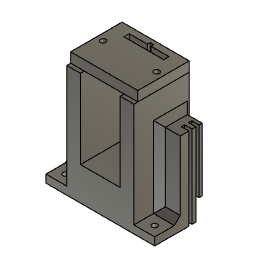
NeckServoMount v8 (Autodesk Fusion 360 design; units mm, degrees)
Autodesk Fusion 360 part; units mm, degrees
sketch "Base" plane through (0, 0, 0) normal (0, 0, 1) x (1, 0, 0) in component "NeckServoMount"
  line L0 (0, 0) -> (55.4, 0)
  line L1 (55.4, 0) -> (55.4, 24.2)
  line L2 (55.4, 24.2) -> (0, 24.2)
  line L3 (0, 24.2) -> (0, 0)
  line L4 (0, 13) -> (55.4, 13)
  line L5 (0, 19) -> (55.4, 19) construction
  line L6 (0, 17.4) -> (55.4, 17.4) construction
  line L7 (0, 21) -> (55.4, 21) construction
  line L8 (0, 22.6) -> (55.4, 22.6) construction
  line L9 (3.8, 22.6) -> (3.8, 21)
  line L10 (3.8, 19) -> (3.8, 17.4)
  line L11 (0, 22.6) -> (3.8, 22.6)
  line L12 (3.8, 21) -> (0, 21)
  line L13 (0, 19) -> (3.8, 19)
  line L14 (0, 17.4) -> (3.8, 17.4)
  line L15 (27.7, 24.2) -> (27.7, 0) construction
  line L16 (55.4, 22.6) -> (51.6, 22.6)
  line L17 (51.6, 22.6) -> (51.6, 21)
  line L18 (51.6, 21) -> (55.4, 21)
  line L19 (51.6, 19) -> (51.6, 17.4)
  line L20 (55.4, 19) -> (51.6, 19)
  line L21 (55.4, 17.4) -> (51.6, 17.4)
  dimension "d1" = 55.4
  dimension "d3" = 13
  dimension "d4" = 4.4
  dimension "d5" = 1.6
  dimension "d6" = 2
  dimension "d7" = 1.6
  dimension "d8" = 1.6
  dimension "d9" = 3.8
  constraint horizontal L0
  constraint vertical L1
  constraint horizontal L2
  constraint vertical L3
  constraint coincident L0.start L3.end
  constraint coincident L3 L4.start
  constraint coincident L1 L4.end
  constraint perpendicular L1 L4
  constraint coincident L3 L5.start
  constraint coincident L1 L5.end
  constraint perpendicular L1 L5
  constraint coincident L3 L6.start
  constraint coincident L1 L6.end
  constraint perpendicular L1 L6
  constraint coincident L3 L7.start
  constraint coincident L1 L7.end
  constraint perpendicular L1 L7
  constraint coincident L3 L8.start
  constraint coincident L1 L8.end
  constraint perpendicular L1 L8
  constraint coincident L8 L9.start
  constraint coincident L7 L9.end
  constraint perpendicular L7 L9
  constraint coincident L5 L10.start
  constraint coincident L6 L10.end
  constraint perpendicular L6 L10
  constraint collinear L9 L10
  constraint midpoint L2 L15.start
  constraint midpoint L0 L15.end
  constraint symmetric L5.start L15 L5.end
  constraint symmetric L6.start L15 L6.end
  constraint symmetric L7.start L15 L7.end
  constraint symmetric L8.start L15 L8.end
  constraint symmetric L9.start L15 L16.end
  constraint symmetric L9.end L15 L17.end
  constraint symmetric L10.start L15 L19.start
  constraint symmetric L10.end L15 L19.end
  measures "d1" distance of L0.start L0.end
  measures "d3" distance of L0 L4
  measures "d4" distance of L4 L6
  measures "d5" distance of L5 L6
  measures "d6" distance of L5 L7
  measures "d7" distance of L7 L8
  measures "d8" distance of L2 L8
  measures "d9" distance of L3 L9
extrude "ExtrudeSlottedVertical" add sketch "Base" along normal blind 42 contours L1 L2 L3 L4 L9 L10 L11 L12 L13 L14 L16 L17 L18 L19 L20 L21 makes body 1 in component "NeckServoMount"
extrude "ExtrudeBasePlate" add sketch "Base" along normal blind 4 contours L0 L1 L3 L4 bodies 1 in component "NeckServoMount"
sketch "Back" plane through (0, 24.2, 0) normal (0, 1, 0) x (-1, 0, 0) in component "NeckServoMount"
  line L0 (-55.4, 0) -> (0, 0)
  line L1 (0, 0) -> (0, 42)
  line L2 (0, 42) -> (-55.4, 42)
  line L3 (-55.4, 42) -> (-55.4, 0)
  line L4 (-55.4, 0) -> (0.6, 0)
  line L5 (0.6, 0) -> (0.6, 10)
  line L6 (0.6, 10) -> (-55.4, 10)
  line L7 (-55.4, 10) -> (-55.4, 0)
  dimension "d19" = 10
  constraint horizontal L4
  constraint vertical L5
  constraint horizontal L6
  constraint vertical L7
  constraint coincident L0.start L3.end
  measures "d19" distance of L0.start L6.end
extrude "CutBackAway" cut sketch "Back" against normal up to surface (3.2 mm away) contours L0 L1 L3 L4 L6 L7 bodies 1 in component "NeckServoMount"
chamfer "Chamfer1" distance 3 angle 45 1 edges at (27.7, 13, 4) on bodies 1 in component "NeckServoMount"
sketch "ScrewHoles" plane through (0, 0, 4) normal (0, 0, 1) x (-1, 0, 0) in component "NeckServoMount"
  line L0 (-55.4, -10) -> (0, -10)
  line L1 (0, -10) -> (0, 0)
  line L2 (0, 0) -> (-55.4, 0)
  line L3 (-55.4, 0) -> (-55.4, -10)
  line L4 (0, -5) -> (-55.4, -5) construction
  circle A0 centre (-5, -5) radius 1.4
  line L5 (-27.7, 0) -> (-27.7, -10) construction
  circle A1 centre (-50.4, -5) radius 1.4
  dimension "d23" = 2.8
  dimension "d49" = 5
  constraint midpoint L1 L4.start
  constraint midpoint L3 L4.end
  constraint coincident L4 A0.centre
  constraint midpoint L2 L5.start
  constraint midpoint L0 L5.end
  constraint symmetric A0 L5 A1
  measures "d23" diameter of A0
  measures "d49" distance of L1 A0.centre
extrude "CutScrewHoles" cut sketch "ScrewHoles" against normal up to surface (4 mm away) contours A0 | A1 bodies 1 in component "NeckServoMount"
sketch "ServoU" plane through (0, 24.2, 0) normal (0, 1, 0) x (-1, 0, 0) in component "NeckServoMount"
  line L0 (-55.4, 10) -> (0, 10)
  line L1 (0, 10) -> (0, 42)
  line L2 (0, 42) -> (-55.4, 42)
  line L3 (-55.4, 42) -> (-55.4, 10)
  line L4 (0, 0) -> (-55.4, 0)
  line L5 (-37.8, 57.2) -> (-17.6, 57.2)
  line L6 (-17.6, 57.2) -> (-17.6, 17)
  line L7 (-17.6, 17) -> (-37.8, 17)
  line L8 (-37.8, 17) -> (-37.8, 57.2)
  line L9 (-10.6, 57.2) -> (-10.6, 3)
  line L10 (-44.8, 57.2) -> (-44.8, 3)
  line L11 (-44.8, 3) -> (-10.6, 3)
  line L12 (-10.6, 57.2) -> (-17.6, 57.2)
  line L13 (-37.8, 57.2) -> (-44.8, 57.2)
  point P0 (-10.6, 57.2)
  point P1 (-44.8, 57.2)
  dimension "d26" = 20.2
  dimension "d27" = 40.2
  dimension "d29" = 17.6
  dimension "d31" = 17
  dimension "d34" = 7
  dimension "d35" = 7
  dimension "d36" = 14
  constraint horizontal L5
  constraint vertical L6
  constraint horizontal L7
  constraint vertical L8
  constraint horizontal L5.start P1
  constraint horizontal P0 P1
  constraint coincident P0 L9.start
  constraint perpendicular L4 L9
  constraint coincident P1 L10.start
  constraint perpendicular L4 L10
  constraint horizontal L9.end L10.end
  measures "d26" distance of L5.start L5.end
  measures "d27" distance of L5.start L7.end
  measures "d29" distance of L3 L8
  measures "d31" distance of L4 L7
  measures "d34" distance of L8 P1
  measures "d35" distance of L6 P0
  measures "d36" distance of L7 L11
extrude "ExtrudeServoU" add sketch "ServoU" against normal up to surface (22.2 mm away) from surface at -2 contours L0 L2 L6 L7 L8 L9 L10 | L0 L9 L10 L11 | L2 L8 L10 L13 | L2 L6 L9 L12 bodies 1 in component "NeckServoMount"
extrude "CutServoU" cut sketch "ServoU" against normal blind 2 contours L0 L2 L6 L7 L8 L9 L10 | L0 L9 L10 L11 | L2 L8 L10 L13 | L2 L6 L9 L12 bodies 1 in component "NeckServoMount"
extrude "CutServoU2" cut sketch "ServoU" against normal through all contours L2 L5 L6 L8 | L2 L6 L7 L8 bodies 1 in component "NeckServoMount"
extrude "CutBackAwayAgain" cut sketch "Back" against normal up to surface (3.2 mm away) contours L0 L1 L3 L4 L6 L7 bodies 1 in component "NeckServoMount"
sketch "BottomSlot" plane through (0, 0, 17) normal (0, 0, 1) x (-1, 0, 0) in component "NeckServoMount"
  line L0 (-17.6, -22.2) -> (-17.6, 0)
  line L1 (-17.6, 0) -> (-37.8, 0)
  line L2 (-37.8, 0) -> (-37.8, -22.2)
  line L3 (-37.8, -22.2) -> (-17.6, -22.2)
  line L4 (-17.6, -22.2) -> (-37.8, -22.2)
  line L5 (-37.8, -22.2) -> (-37.8, -24.9)
  line L6 (-37.8, -24.9) -> (-17.6, -24.9)
  line L7 (-17.6, -24.9) -> (-17.6, -22.2)
  dimension "d54" = 2.7
  dimension "d55" = 20.2
  constraint horizontal L4
  constraint vertical L5
  constraint horizontal L6
  constraint vertical L7
  constraint coincident L0.start L3.end
  measures "d54" distance of L0.start L6.end
  measures "d55" distance of L5 L7
extrude "ExtrudeSlotHolder" add 1 faces at (15.2667, 22.2, 38.7333) along direction (0, 1, 0) blind 6 on bodies 1 bodies 1 in component "NeckServoMount"
extrude "CutBottomSlot" cut sketch "BottomSlot" against normal up to surface (7 mm away) contours L3 L4 L5 L6 L7 bodies 1 in component "NeckServoMount"
sketch "TinySlot" plane through (0, 24.9, 0) normal (0, -1, 0) x (1, 0, 0)
  line L0 (17.6, 10) -> (37.8, 10)
  line L1 (37.8, 10) -> (37.8, 17)
  line L2 (37.8, 17) -> (17.6, 17)
  line L3 (17.6, 17) -> (17.6, 10)
  line L4 (26.8, 17) -> (28.6, 17)
  line L5 (28.6, 17) -> (28.6, 10)
  line L6 (28.6, 10) -> (26.8, 10)
  line L7 (26.8, 10) -> (26.8, 17)
  point P0 (27.7, 17)
  point P1 (27.7, 17)
  dimension "d61" = 1.8
  dimension "d62" = 7
  constraint horizontal L4
  constraint vertical L5
  constraint horizontal L6
  constraint vertical L7
  constraint coincident L2 L4.start
  constraint midpoint L2 P1
  constraint midpoint L4 P1
  constraint coincident P1 P0
  measures "d61" distance of L4.start L4.end
  measures "d62" distance of L4.start L6.end
extrude "CutTinySlot" cut sketch "TinySlot" against normal blind 1.4 contours L0 L2 L4 L5 L6 L7 bodies 1 in component "NeckServoMount"
sketch "TopPlate" plane through (0, 0, 57.2) normal (0, 0, 1) x (-1, 0, 0) in component "TopPlate"
  line L0 (-10.6, 0) -> (-17.6, 0)
  line L1 (-17.6, 0) -> (-17.6, -28.2)
  line L2 (-17.6, -28.2) -> (-10.6, -28.2)
  line L3 (-10.6, -28.2) -> (-10.6, 0)
  line L4 (-10.6, -28.2) -> (-44.8, -28.2)
  line L5 (-44.8, -28.2) -> (-44.8, -2)
  line L6 (-44.8, -2) -> (-10.6, -2)
  line L7 (-10.6, -2) -> (-10.6, -28.2)
  line L8 (-44.8, -10) -> (-44.8, 0)
  line L9 (-17.6, -24.9) -> (-26.8, -24.9)
  line L10 (-37.8, -22.2) -> (-17.6, -22.2)
  line L11 (-26.8, -24.9) -> (-26.8, -26.3)
  line L12 (-26.8, -26.3) -> (-28.6, -26.3)
  line L13 (-28.6, -26.3) -> (-28.6, -24.9)
  line L14 (-28.6, -24.9) -> (-37.8, -24.9)
  line L15 (-37.8, -24.9) -> (-37.8, -28.2)
  line L16 (-37.8, -28.2) -> (-17.6, -28.2)
  line L17 (-17.6, -28.2) -> (-17.6, -24.9)
  line L18 (-17.6, -24.9) -> (-26.8, -24.9)
  line L19 (-37.8, 0) -> (-37.8, -28.2)
  line L20 (-17.6, -22.2) -> (-37.8, -22.2)
  dimension "d66" = 2
  constraint horizontal L4
  constraint vertical L5
  constraint horizontal L6
  constraint vertical L7
  constraint coincident L5.end L8
  constraint coincident L2.end L3.start
  measures "d66" distance of L0 L6
extrude "ExtrudeTopPlate" add sketch "TopPlate" along normal blind 5 separate body contours L1 L2 L3 L4 L6 L7 L17 | L1 L6 L10 L19 L20 | L4 L5 L6 L8 L15 L19 | L1 L4 L9 L11 L12 L13 L14 L15 L16 L17 L18 L19 makes body 2 in component "TopPlate"
sketch "ScrewHoles (2)" plane through (0, 0, 62.2) normal (0, 0, 1) x (-1, 0, 0) in component "TopPlate"
  line L0 (-17.6, -22.2) -> (-17.6, -24.9)
  line L1 (-17.6, -24.9) -> (-26.8, -24.9)
  line L2 (-26.8, -24.9) -> (-26.8, -26.3)
  line L3 (-26.8, -26.3) -> (-28.6, -26.3)
  line L4 (-28.6, -26.3) -> (-28.6, -24.9)
  line L5 (-28.6, -24.9) -> (-37.8, -24.9)
  line L6 (-37.8, -24.9) -> (-37.8, -22.2)
  line L7 (-37.8, -22.2) -> (-17.6, -22.2)
  line L8 (-44.8, -28.2) -> (-10.6, -28.2)
  line L9 (-10.6, -28.2) -> (-10.6, -2)
  line L10 (-10.6, -2) -> (-44.8, -2)
  line L11 (-44.8, -2) -> (-44.8, -28.2)
  line L12 (-37.8, 0) -> (-44.8, 0)
  line L13 (-37.8, -28.2) -> (-44.8, -28.2) construction
  line L14 (-41.3, -28.2) -> (-41.3, 0) construction
  line L15 (-41.3, -28.2) -> (-41.3, -2) construction
  circle A0 centre (-41.3, -15.1) radius 1.4
  line L16 (-27.7, -2) -> (-27.7, -28.2) construction
  circle A1 centre (-14.1, -15.1) radius 1.4
  point P0 (-41.3, 0)
  point P1 (-41.3, -28.2)
  point P2 (-41.3, -2)
  point P3 (-41.3, -15.1)
  dimension "d69" = 2.8
  constraint midpoint P0 L12
  constraint midpoint P1 L13
  constraint coincident P1 L14.start
  constraint coincident P0 L14.end
  constraint coincident L10 P2
  constraint coincident L14 P2
  constraint coincident P2 L15.end
  constraint midpoint L15 P3
  constraint coincident P3 A0.centre
  constraint midpoint L10 L16.start
  constraint midpoint L8 L16.end
  constraint symmetric A0 L16 A1
  measures "d69" diameter of A0
extrude "CutHoles" cut sketch "ScrewHoles (2)" against normal blind 13 contours A0 | A1 bodies 1 in component "NeckServoMount"
extrude "Extrude2" cut sketch "ScrewHoles (2)" against normal blind 13 contours A0 | A1 bodies 2 in component "TopPlate"
chamfer "Chamfer3" distance 3 angle 45 6 edges at (44.8, 13, 24.5) (10.6, 13, 24.5) (10.6, 24.2, 26) (44.8, 24.2, 26) (10.6, 18.6, 42) (44.8, 18.6, 42) on bodies 1 in component "NeckServoMount"
component "NeckServoMount" placed x (1, 0, 0) y (0, 1, 0) z (0, 0, 1) at (0, 0, 0)
component "TopPlate" placed x (1, 0, 0) y (0, 1, 0) z (0, 0, 1) at (0, 0, 0)
equation "servo_offset_x = 17.6 mm"
equation "d29 = servo_offset_x"
equation "servo_offset_z = 17 mm"
equation "d31 = servo_offset_z"
equation "servo_offset_y = 2 mm"
equation "d38 = -servo_offset_y"
equation "d41 = -servo_offset_y"
named bodies: "NeckServoMount", "TopPlate"
